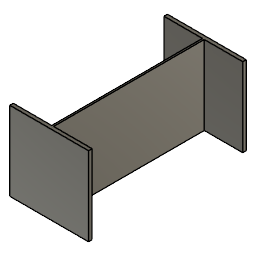
軽H-200×100×2.3×4.5 (Autodesk Fusion 360 design; units mm, degrees)
Autodesk Fusion 360 part; units mm, degrees
sketch "スケッチ1" plane through (0, 0, 0) normal (0, 0, 1) x (1, 0, 0)
  line L0 (0, -95.5) -> (0, 95.5)
  line L1 (-50, 100) -> (50, 100)
  line L2 (-50, -100) -> (50, -100)
  line L3 (1.15, -95.5) -> (1.15, 95.5)
  line L4 (-1.15, -95.5) -> (-1.15, 95.5)
  line L5 (-50, -95.5) -> (-1.15, -95.5)
  line L6 (1.15, -95.5) -> (50, -95.5)
  line L7 (-50, 95.5) -> (-1.15, 95.5)
  line L8 (1.15, 95.5) -> (50, 95.5)
  line L9 (50, 100) -> (50, 95.5)
  line L10 (-50, 100) -> (-50, 95.5)
  line L11 (-50, -95.5) -> (-50, -100)
  line L12 (50, -95.5) -> (50, -100)
  dimension "d2" = 100
  dimension "d3" = 100
  constraint vertical L0
  constraint horizontal L1
  constraint perpendicular L0 L2
  constraint coincident L3.start L5
  constraint coincident L0.start L5
  constraint coincident origin L0
  constraint collinear L5 L6
  constraint coincident L3.end L7
  constraint coincident L0.end L7
  constraint collinear L7 L8
  constraint perpendicular L1 L9
  constraint perpendicular L1 L10
  constraint perpendicular L2 L11
  constraint perpendicular L2 L12
  measures "d2" distance of L1.start L1.end
  measures "d3" distance of L2.start L2.end
extrude "押し出し1" add sketch "スケッチ1" along normal blind 100
